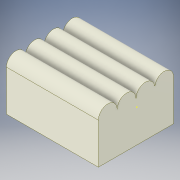
# Autodesk Inventor part: Battery Box
Saved by Autodesk Inventor 2018 (Build 220112000, 112)
## iProperties
Created: 2018-02-19
Part Number: Battery Box
Material: Generic
Document SubType Name: Modeling
Designer: Melda
Density: 1 g/cm^3
Appearance: Smooth - Ivory
Author: Melda
Autodesk Inventor part; units mm, degrees
ref_plane "YZ Plane" through (0, 0, 0) normal (1, 0, 0) x (0, 1, 0)
ref_plane "XZ Plane" through (0, 0, 0) normal (0, 1, 0) x (-1, 0, 0)
ref_plane "XY Plane" through (0, 0, 0) normal (0, 0, 1) x (1, 0, 0)
sketch "Sketch1" plane through (0, 0, 0) normal (1, 0, 0) x (0, 1, 0)
  point P0 (0, 0)
sketch "Sketch2" plane through (0, 0, 0) normal (1, 0, 0) x (0, 1, 0)
  line L0 (10.2809, 22.9213) -> (-19.7191, 22.9213)
  line L1 (-19.7191, 22.9213) -> (-19.7191, -22.0787)
  line L2 (-19.7191, -22.0787) -> (10.2809, -22.0787)
  line L3 (10.2809, -22.0787) -> (10.2809, 22.9213)
  point P0 (0, 0)
  dimension "d0" = 45
  dimension "d1" = 30
  constraints: 8 end point, 2 parallel, 1 horizontal, 1 perpendicular
  measures "d0" distance of L2.end L0.start
  measures "d1" distance of L1.end L2.end
extrude "Extrusion1" add sketch "Sketch2" along normal blind 55
sketch "Sketch3" plane through (55, 0, 0) normal (1, 0, 0) x (0, 0, -1)
  point P0 (0, 0)
sketch "Sketch4" plane through (55, 0, 0) normal (1, 0, 0) x (0, 0, -1)
  arc A0 (-11.6713, 4.6559) -> (-22.9213, 4.6559) centre (-17.2963, 4.6559) ccw
  line L0 (-22.9213, 10.2809) -> (-22.9213, -19.7191) projected
  line L1 (22.0787, 10.2809) -> (-22.9213, 10.2809) projected
  arc A1 (-0.3979, 4.6559) -> (-11.6479, 4.6559) centre (-6.0229, 4.6559) ccw
  arc A2 (10.7927, 5.4828) -> (-0.3962, 4.6559) centre (5.2288, 4.6559) ccw
  arc A3 (22.0731, 4.6559) -> (10.8842, 5.4828) centre (16.4481, 4.6559) ccw
  line L2 (-22.9213, 4.6559) -> (-22.9213, 10.2809)
  line L3 (-22.9213, 10.2809) -> (22.0787, 10.2809)
  line L4 (22.0787, 10.2809) -> (22.0787, 4.6559)
  line L5 (22.0787, -19.7191) -> (22.0787, 10.2809) projected
  line L6 (10.7927, 5.4828) -> (10.8842, 5.4828)
  line L7 (-22.9213, 4.6559) -> (22.0787, 4.6559)
  point P0 (0, 0)
  dimension "d4" = 11.25
  dimension "d5" = 11.25
  dimension "d6" = 11.25
  dimension "d7" = 11.25
  constraints: 10 end point, 8 point on circle, 7 point on line, 4 centre point, 3 tangent, 2 collinear, 2 horizontal
  measures "d4" diameter of A0
  measures "d5" diameter of A1
  measures "d6" diameter of A2
  measures "d7" diameter of A3
extrude "Extrusion2" cut sketch "Sketch4" against normal blind 60 contours A0 L1 A1 L7 | A0 L0 L1 | L1 A2 A1 | L1 A3 L6 A2 | A3 L1 L4 L7
body "Solid1"
